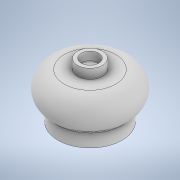
# Autodesk Inventor part: 77. Колпак защитный
Saved by Autodesk Inventor 2021 (Build 250183000, 183)
## iProperties
Created: 2021-03-19
Part Number: 77. Колпак защитный
Material: Типовые
Document SubType Name: Modeling
Designer: Данил
Density: 1 g/cm^3
Appearance: По умолчанию
Author: Данил
Autodesk Inventor part; units mm, degrees
ref_plane "YZ Plane" through (0, 0, 0) normal (1, 0, 0) x (0, 1, 0)
ref_plane "XZ Plane" through (0, 0, 0) normal (0, 1, 0) x (-1, 0, 0)
ref_plane "XY Plane" through (0, 0, 0) normal (0, 0, 1) x (1, 0, 0)
sketch "Эскиз1" plane through (0, 0, 0) normal (0, 0, 1) x (1, 0, 0)
  line L0 (0, 30) -> (0, -30)
  line L1 (30.5, -30) -> (35, -30)
  line L2 (35, -30) -> (35, -15.8955)
  line L3 (30.5, -30) -> (30.5, -15.6635)
  arc A0 (32.3947, -12.8745) -> (26.5, 18) centre (26.5, 2) ccw
  arc A1 (36.5366, -13.2767) -> (28, 19.5) centre (28, 2) ccw
  line L4 (26.5, 18) -> (12.5, 18)
  line L5 (28, 19.5) -> (13.5, 19.5)
  line L6 (13.5, 19.5) -> (13.5, 30)
  line L7 (9.5, 21) -> (9.5, 30)
  line L8 (9.5, 30) -> (13.5, 30)
  arc A2 (9.5, 21) -> (12.5, 18) centre (12.5, 21) ccw
  arc A3 (36.5366, -13.2767) -> (35, -15.8955) centre (38, -15.8955) ccw
  arc A4 (32.3947, -12.8745) -> (30.5, -15.6635) centre (33.5, -15.6635) ccw
  point P0 (0, 0)
  point P1 (0, 0)
  point P2 (35, -14.039)
  point P3 (30.5, -13.4919)
  dimension "d0" = 60
  dimension "d1" = 61
  dimension "d2" = 70
  dimension "d3" = 16
  dimension "d4" = 1.5
  dimension "d5" = 32
  dimension "d6" = 19
  dimension "d7" = 27
  dimension "d8" = 53
  dimension "d10" = 1.5
  dimension "d11" = 3
  dimension "d12" = 3
  constraints: 18 end point, 12 point on circle, 8 tangent, 5 centre point, 3 horizontal, 3 horizontal alignment, 3 perpendicular, 3 vertical, 2 point on line, 1 coincident, 1 equal radius, 1 midpoint
  measures "d0" distance of L0.start L0.end
  measures "d1" diameter of L3 L0
  measures "d2" diameter of L2 L0
  measures "d3" radius of A0
  measures "d4" distance of A0.centre A1.centre
  measures "d5" vertical distance of L0.end A1.centre
  measures "d6" diameter of L7 L0
  measures "d7" diameter of L6 L0
  measures "d8" diameter of A0.centre L0
  measures "d10" distance between parallel lines of L4 L5
  measures "d11" radius of A2
  measures "d12" radius of A4
revolve "Вращение1" add sketch "Эскиз1" angle 360 about axis through (0, 30, 0) along (0, -1, 0)
